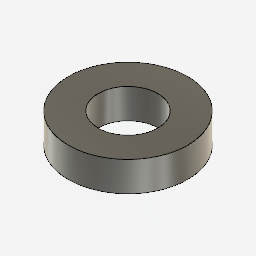
SAE_Washer (Autodesk Fusion 360 design; units mm, degrees)
Autodesk Fusion 360 part; units mm, degrees
sketch "Sketch1" plane through (0, 0, 0) normal (0, 0, 1) x (1, 0, 0)
  circle A0 centre (0, 0) radius 6.35
  circle A1 centre (0, 0) radius 12.7
  dimension "outerdiameter" = 25.4
  dimension "diameter" = 12.7
  measures "outerdiameter" diameter of A1
  measures "diameter" diameter of A0
extrude "Extrude1" add sketch "Sketch1" along normal blind 6.35
equation "thickness = 0.25 in"
